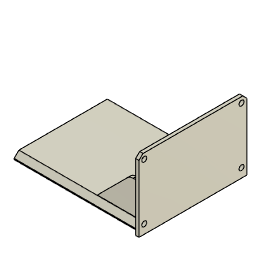
CPU Tray - Template (Autodesk Fusion 360 design; units mm, degrees)
Autodesk Fusion 360 part; units mm, degrees
sketch "sketch 1797" plane through (92, 0, 0) normal (1, 0, 0) x (0, 1, 0)
  circle A0 centre (-79.085, 49.8044) radius 1.8
  circle A1 centre (-79.085, 9.5044) radius 1.8
  circle A2 centre (-9.085, 9.5044) radius 1.8
  circle A3 centre (-9.085, 49.8044) radius 1.8
  line L0 (-17.15, 13.7) -> (-34.35, 13.7)
  line L1 (-34.35, 13.7) -> (-34.35, 28.7)
  line L2 (-34.35, 28.7) -> (-17.15, 28.7)
  line L3 (-17.15, 28.7) -> (-17.15, 13.7)
  line L4 (-70, 14.5) -> (-70, 29.9)
  line L5 (-70, 29.9) -> (-69.9878, 30.0389)
  line L6 (-69.9878, 30.0389) -> (-69.9518, 30.1736)
  line L7 (-69.9518, 30.1736) -> (-69.8928, 30.3)
  line L8 (-69.8928, 30.3) -> (-69.8128, 30.4142)
  line L9 (-69.8128, 30.4142) -> (-69.7142, 30.5128)
  line L10 (-69.7142, 30.5128) -> (-69.6, 30.5928)
  line L11 (-69.6, 30.5928) -> (-69.4736, 30.6518)
  line L12 (-69.4736, 30.6518) -> (-69.3389, 30.6878)
  line L13 (-69.3389, 30.6878) -> (-69.2, 30.7)
  line L14 (-69.2, 30.7) -> (-55.8, 30.7)
  line L15 (-55.8, 30.7) -> (-55.6611, 30.6878)
  line L16 (-55.6611, 30.6878) -> (-55.5264, 30.6518)
  line L17 (-55.5264, 30.6518) -> (-55.4, 30.5928)
  line L18 (-55.4, 30.5928) -> (-55.2858, 30.5128)
  line L19 (-55.2858, 30.5128) -> (-55.1872, 30.4142)
  line L20 (-55.1872, 30.4142) -> (-55.1072, 30.3)
  line L21 (-55.1072, 30.3) -> (-55.0482, 30.1736)
  line L22 (-55.0482, 30.1736) -> (-55.0122, 30.0389)
  line L23 (-55.0122, 30.0389) -> (-55, 29.9)
  line L24 (-55, 29.9) -> (-55, 14.5)
  line L25 (-55, 14.5) -> (-55.0122, 14.3611)
  line L26 (-55.0122, 14.3611) -> (-55.0482, 14.2264)
  line L27 (-55.0482, 14.2264) -> (-55.1072, 14.1)
  line L28 (-55.1072, 14.1) -> (-55.1872, 13.9858)
  line L29 (-55.1872, 13.9858) -> (-55.2858, 13.8872)
  line L30 (-55.2858, 13.8872) -> (-55.4, 13.8072)
  line L31 (-55.4, 13.8072) -> (-55.5264, 13.7482)
  line L32 (-55.5264, 13.7482) -> (-55.6611, 13.7122)
  line L33 (-55.6611, 13.7122) -> (-55.8, 13.7)
  line L34 (-55.8, 13.7) -> (-69.2, 13.7)
  line L35 (-69.2, 13.7) -> (-69.3389, 13.7122)
  line L36 (-69.3389, 13.7122) -> (-69.4736, 13.7482)
  line L37 (-69.4736, 13.7482) -> (-69.6, 13.8072)
  line L38 (-69.6, 13.8072) -> (-69.7142, 13.8872)
  line L39 (-69.7142, 13.8872) -> (-69.8128, 13.9858)
  line L40 (-69.8128, 13.9858) -> (-69.8928, 14.1)
  line L41 (-69.8928, 14.1) -> (-69.9518, 14.2264)
  line L42 (-69.9518, 14.2264) -> (-69.9878, 14.3611)
  line L43 (-69.9878, 14.3611) -> (-70, 14.5)
  line L44 (-52, 14.5) -> (-52, 29.9)
  line L45 (-52, 29.9) -> (-51.9878, 30.0389)
  line L46 (-51.9878, 30.0389) -> (-51.9518, 30.1736)
  line L47 (-51.9518, 30.1736) -> (-51.8928, 30.3)
  line L48 (-51.8928, 30.3) -> (-51.8128, 30.4142)
  line L49 (-51.8128, 30.4142) -> (-51.7142, 30.5128)
  line L50 (-51.7142, 30.5128) -> (-51.6, 30.5928)
  line L51 (-51.6, 30.5928) -> (-51.4736, 30.6518)
  line L52 (-51.4736, 30.6518) -> (-51.3389, 30.6878)
  line L53 (-51.3389, 30.6878) -> (-51.2, 30.7)
  line L54 (-51.2, 30.7) -> (-37.8, 30.7)
  line L55 (-37.8, 30.7) -> (-37.6611, 30.6878)
  line L56 (-37.6611, 30.6878) -> (-37.5264, 30.6518)
  line L57 (-37.5264, 30.6518) -> (-37.4, 30.5928)
  line L58 (-37.4, 30.5928) -> (-37.2858, 30.5128)
  line L59 (-37.2858, 30.5128) -> (-37.1872, 30.4142)
  line L60 (-37.1872, 30.4142) -> (-37.1072, 30.3)
  line L61 (-37.1072, 30.3) -> (-37.0482, 30.1736)
  line L62 (-37.0482, 30.1736) -> (-37.0122, 30.0389)
  line L63 (-37.0122, 30.0389) -> (-37, 29.9)
  line L64 (-37, 29.9) -> (-37, 14.5)
  line L65 (-37, 14.5) -> (-37.0122, 14.3611)
  line L66 (-37.0122, 14.3611) -> (-37.0482, 14.2264)
  line L67 (-37.0482, 14.2264) -> (-37.1072, 14.1)
  line L68 (-37.1072, 14.1) -> (-37.1872, 13.9858)
  line L69 (-37.1872, 13.9858) -> (-37.2858, 13.8872)
  line L70 (-37.2858, 13.8872) -> (-37.4, 13.8072)
  line L71 (-37.4, 13.8072) -> (-37.5264, 13.7482)
  line L72 (-37.5264, 13.7482) -> (-37.6611, 13.7122)
  line L73 (-37.6611, 13.7122) -> (-37.8, 13.7)
  line L74 (-37.8, 13.7) -> (-51.2, 13.7)
  line L75 (-51.2, 13.7) -> (-51.3389, 13.7122)
  line L76 (-51.3389, 13.7122) -> (-51.4736, 13.7482)
  line L77 (-51.4736, 13.7482) -> (-51.6, 13.8072)
  line L78 (-51.6, 13.8072) -> (-51.7142, 13.8872)
  line L79 (-51.7142, 13.8872) -> (-51.8128, 13.9858)
  line L80 (-51.8128, 13.9858) -> (-51.8928, 14.1)
  line L81 (-51.8928, 14.1) -> (-51.9518, 14.2264)
  line L82 (-51.9518, 14.2264) -> (-51.9878, 14.3611)
  line L83 (-51.9878, 14.3611) -> (-52, 14.5)
  line L84 (-8.1678, 53.8044) -> (-80.0022, 53.8044)
  line L85 (-80.0022, 53.8044) -> (-82.885, 50.9215)
  line L86 (-82.885, 50.9215) -> (-82.885, 3.0044)
  line L87 (-82.885, 3.0044) -> (-76.085, 3.0044)
  line L88 (-76.085, 3.0044) -> (-8.635, 3)
  line L89 (-8.635, 3) -> (-5.285, 3.0041)
  line L90 (-5.285, 3.0044) -> (-5.285, 3.0041)
  line L91 (-5.285, 50.9215) -> (-5.285, 3.0044)
  line L92 (-8.1678, 53.8044) -> (-5.285, 50.9215)
extrude "Extrude1" add sketch "sketch 1797" along normal blind -1.5 and the other way blind -0.9 contours L0 L1 L2 L3 | L4 L5 L6 L7 L8 L9 L10 L11 L12 L13 L14 L15 L16 L17 L18 L19 L20 L21 L22 L23 L24 L25 L26 L27 L28 L29 L30 L31 L32 L33 L34 L35 L36 L37 L38 L39 L40 L41 L42 L43 | L44 L45 L46 L47 L48 L49 L50 L51 L52 L53 L54 L55 L56 L57 L58 L59 L60 L61 L62 L63 L64 L65 L66 L67 L68 L69 L70 L71 L72 L73 L74 L75 L76 L77 L78 L79 L80 L81 L82 L83 | L84 L85 L86 L87 L88 L89 L91 L92
sketch "sketch 1545" plane through (92, 0, 0) normal (1, 0, 0) x (0, 1, 0)
  line L0 (-12.285, 7.1672) -> (-75.885, 7.1672)
  line L1 (-75.885, 7.1672) -> (-79.335, 3.7172)
  line L2 (-79.335, 3.7172) -> (-79.335, 3.0044)
  line L3 (-79.335, 3.0044) -> (-76.085, 3.0044)
  line L4 (-76.085, 3.0044) -> (-8.835, 3)
  line L5 (-8.835, 3) -> (-8.835, 3.7172)
  line L6 (-8.835, 3.7172) -> (-12.285, 7.1672)
extrude "Extrude2" add sketch "sketch 1545" against normal up to surface (92.5 mm away)
ref_plane "WorkPlane1" through (91.7, -75.685, 26.963) normal (0, -1, 0) x (0, 0, 1)
sketch "Sketch1" plane through (91.25, -75.685, 27.0044) normal (0, -1, 0) x (0, 0, 1)
  line L0 (26.8, 0.75) -> (-19.8372, 0.75)
  line L1 (-19.8372, 91.75) -> (-24, 91.75)
  line L2 (-24, 91.75) -> (-24, -1.65)
  line L3 (-24, -1.65) -> (26.8, -1.65)
  line L4 (1.7619, 13.9501) -> (-19.8562, 35.5682)
  line L5 (26.8, 0.75) -> (-39.2378, 0.75) construction
  line L6 (3.5193, 9.682) -> (3.4814, 0.75)
  arc A0 (3.5193, 9.682) -> (1.7619, 13.9501) centre (-2.4807, 9.7074) ccw
  line L7 (26.8, -1.65) -> (26.8, 0.75)
  line L8 (-19.8372, 0.75) -> (-19.8372, 91.75)
  dimension "d614" = 45
  dimension "d615" = 6
  constraint horizontal L5
  constraint coincident L0.start L5.start
  constraint midpoint L0 L6.end
  constraint tangent L4 A0
  constraint tangent L6 A0
  measures "d614" angle of L4 L5
  measures "d615" radius of A0
extrude "Extrude8" add sketch "Sketch1" against normal blind 2.4 contours L0 L4 L6 A0 L8
extrude "Extrude9" add 1 faces at (74.5002, -75.685, 14.3669) along direction (0, -1, 0) blind 2.4 from surface at -63.2
